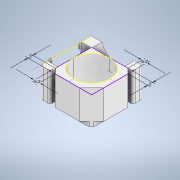
# Autodesk Inventor part: xy-mount-bottom-copy
Saved by Autodesk Inventor 2020 (Build 240168000, 168)
## iProperties
Created: 2021-03-01
Part Number: xy-mount-bottom-copy
Material: ABS Plastic
Document SubType Name: Modeling
Designer: AOB
Mass: 2.83472 g
Surface Area: 25.5195 cm^2
Volume: 2.67426 cm^3
Density: 1.06 g/cm^3
Appearance: White
Author: AOB
Autodesk Inventor part; units mm, degrees
ref_plane "YZ Plane" through (0, 0, 0) normal (1, 0, 0) x (0, 1, 0)
ref_plane "XZ Plane" through (0, 0, 0) normal (0, 1, 0) x (-1, 0, 0)
ref_plane "XY Plane" through (0, 0, 0) normal (0, 0, 1) x (1, 0, 0)
sketch "Sketch1" plane through (0, 0, 0) normal (0, 0, 1) x (1, 0, 0)
  line L0 (0, 0) -> (21, 0)
  line L1 (21, 0) -> (21, -24)
  line L2 (21, -24) -> (0, -24)
  line L3 (0, -24) -> (0, 0)
  line L4 (4, 0) -> (4, -24)
  line L5 (0, -24) -> (21, 0) construction
  line L6 (0, 0) -> (10.5, -12) construction
  dimension "d0" = 4
  dimension "d2" = 17
  dimension "d61" = 24
  constraints: 14 end point, 2 midpoint, 2 parallel, 2 perpendicular, 2 point on line, 1 horizontal
  measures "d0" distance of L0.start L4.start
  measures "d2" distance of L0.end L4.start
  measures "d61" distance of L0.end L1.end
extrude "Extrusion1" add sketch "Sketch1" along normal blind 17 contours L0 L4 L2 L3
extrude "Extrusion2" add sketch "Sketch1" against normal blind 4
sketch "Sketch2" plane through (0, 0, 0) normal (0, 0, 1) x (1, 0, 0)
  point P0 (0, 0)
  point P1 (11.0344, -10.0001)
hole "Hole1" at (11.0344, -10.0001, 0) direction (0, 0, -1) diameter 14 end through all
sketch "Sketch3" plane through (4, -24, 17) normal (1, 0, 0) x (0, 0, -1)
  line L0 (11.8812, 10.4951) -> (9.8812, 10.4951)
  point P0 (17, 24)
  constraints: 2 coincident, 2 end point, 4 other
hole "Hole2" at (4, -13.5049, 7.1188) direction (-1, 0, 0) diameter 14 end through all
fillet "Fillet2" radius 1 4 edges at (4, -12, 17) (0, -12, 17) (21, -12, 0) (21, -12, -4)
fillet "Fillet3" radius 0.1 1 edges at (4, -12, 0)
sketch "Sketch5" plane through (0, 0, -4) normal (0, 1, 0) x (1, 0, 0)
  line L0 (4, -4.1188) -> (4, -18.1188) projected
  line L1 (20, -4) -> (4.1, -4) construction
  line L2 (11.5, -4) -> (11.5, -11.5) construction
  line L3 (11.5, -11.5) -> (4, -11.5) construction
  circle A0 centre (11.5, -11.5) radius 7.5
  line L4 (11.5, -11.5) -> (15.8301, -4) construction
  line L5 (19, -11.5) -> (19.6263, -11.5) construction
  line L6 (15.8301, -4) -> (11.5, -4)
  line L7 (11.5, -11.5) -> (7.1699, -4) construction
  line L8 (7.1699, -4) -> (5.0048, -7.75)
  line L9 (11.5, -11.5) -> (2.8397, -11.5) construction
  line L10 (2.8397, -11.5) -> (5.0048, -15.25)
  line L11 (11.5, -11.5) -> (7.1699, -19)
  line L12 (7.1699, -19) -> (11.5, -19)
  line L13 (11.5, -11.5) -> (15.8301, -19) construction
  line L14 (15.8301, -19) -> (17.9952, -15.25)
  line L15 (11.5, -11.5) -> (20.1603, -11.5) construction
  line L16 (20.1603, -11.5) -> (17.9952, -7.75)
  line L17 (20.1603, -11.5) -> (17.9952, -15.25)
  line L18 (15.8301, -4) -> (17.9952, -7.75)
  line L19 (11.5, -4) -> (7.1699, -4)
  line L20 (2.8397, -11.5) -> (5.0048, -7.75)
  line L21 (7.1699, -19) -> (5.0048, -15.25)
  line L22 (15.8301, -19) -> (11.5, -19)
  point P0 (0, -4)
  point P1 (4, -4)
  point P2 (21, -4)
  dimension "d26" = 7.5
  dimension "d27" = 7.5
  dimension "d28" = 60
  dimension "d31" = 360
  constraints: 42 end point, 3 point on line, 3 tangent, 2 perpendicular, 2 point on circle, 1 centre point, 1 coincident, 1 horizontal, 1 parallel, 1 vertical, 31 other
  measures "d26" distance of L2.start L2.end
  measures "d27" distance of L2.end L3.end
  measures "d28" angle of L5 L4
ref_plane "Work Plane1" through (0, -12, -4) normal (0, 1, 0) x (1, 0, 0)
sketch "Sketch6" plane through (0, -12, -4) normal (0, 1, 0) x (1, 0, 0)
  circle A0 centre (11.5, -11.5) radius 7.5 projected
  line L0 (11.5, -19) -> (11.5, -21) construction
  line L1 (19, -11.5) -> (21, -11.5) construction
  line L2 (0, -20) -> (0, 0) projected
  line L3 (0, -25) -> (0, 0) construction
  line L4 (19, -4) -> (4, -4)
  line L5 (4, -4) -> (4, -19)
  line L6 (4, -4.1) -> (4, -20) projected
  line L7 (21, -21) -> (6, -21)
  line L8 (21, -6) -> (21, -21)
  arc A1 (4.1, -4) -> (4, -4.1) centre (4.1, -4.1) ccw projected
  line L9 (21, -6) -> (19, -4)
  line L10 (4, -19) -> (6, -21)
  point P0 (0, -4)
  point P1 (4, -11.5)
  point P2 (4, -11.5)
  point P3 (21, -4)
  point P4 (4, -21)
  point P5 (11.5, -4)
  dimension "d86" = 2
  dimension "d87" = 2
  dimension "d88" = 2
  dimension "d89" = 2
  constraints: 18 end point, 6 point on line, 2 horizontal, 2 point on circle, 1 perpendicular, 1 vertical
  measures "d86" distance of L8.start point (21, -4)
  measures "d87" distance of L4.start point (21, -4)
  measures "d88" distance of L5.end point (4, -21)
  measures "d89" distance of L7.end point (4, -21)
extrude "Extrusion3" add sketch "Sketch6" along normal mid plane 24
sketch "Sketch7" plane through (0, 0, -4) normal (0, 1, 0) x (1, 0, 0)
  circle A0 centre (11.5, -11.5) radius 7.5
  line L0 (4, -4) -> (19, -4)
  line L1 (19, -4) -> (19, -19)
  line L2 (19, -19) -> (4, -19)
  line L3 (4, -19) -> (4, -4)
  circle A1 centre (11.5, -11.5) radius 4.5
  point P0 (4, -11.5)
  point P1 (11.5, -4)
  dimension "d82" = 9
  constraints: 8 end point, 2 centre point, 2 parallel, 1 coincident, 1 horizontal, 1 perpendicular
  measures "d82" diameter of A1
extrude "Extrusion4" add sketch "Sketch7" along normal blind 2 contours A0 | L1 L2 A0 | A0 L0 L1 | L2 L3 A0
mirror "Mirror1" about plane through (0, -12, -4) normal (0, 1, 0) of "Extrusion4"
sketch "Sketch8" plane through (0, -24, -4) normal (-1, 0, 0) x (0, 0, 1)
  line L0 (18.0753, 23) -> (18.0753, -1)
  line L1 (16.4506, 11) -> (16.4506, 10)
  line L2 (16.4506, 10) -> (18.0753, 10)
  line L3 (18.0753, 10) -> (18.0753, 11)
  line L4 (18.0753, 11) -> (18.0753, 12)
  line L5 (16.4506, 12) -> (16.4506, 11)
  line L6 (16.4506, 12) -> (18.0753, 12)
  line L7 (3.1188, 11.5233) -> (3.1188, 9.5233)
  line L8 (3.1188, 9.5233) -> (4.7688, 9.5233)
  line L9 (4.7688, 9.5233) -> (4.7688, 11.5233)
  line L10 (4.7688, 11.5233) -> (3.1188, 11.5233)
  circle A0 centre (11.1188, 10.4951) radius 7 projected
  line L11 (20, 24) -> (20, 0) projected
  line L12 (18.1006, 11) -> (17.4506, 11) construction
  point P0 (4, 24)
  dimension "d44" = 0.65
  dimension "d45" = 1
  dimension "d65" = 0.65
  constraints: 24 end point, 4 perpendicular, 2 parallel, 1 horizontal, 1 midpoint, 1 point on line, 1 vertical, 2 other
  measures "d65" distance of L12.start L12.end
extrude "Extrusion5" add sketch "Sketch8" along normal blind 0.5 contours L0 L2 L1 L5 L6 A0 | A0 L6 L0 | A0 L10 L9 L8 | L8 L7 L10 A0
fillet "Fillet5" radius 2 2 edges at (-0.5, -13.4767, -0.8812) (-0.5, -13, 14.0753)
sketch "Sketch9" plane through (0, 0, -4) normal (0, 0, -1) x (-1, 0, 0)
  circle A0 centre (-11.0344, -10.0001) radius 7 projected
  line L0 (-4.0344, -10.0001) -> (-4.0344, -11.0001)
  line L1 (-4.0344, -11.0001) -> (-3.0344, -11.0001)
  line L2 (-3.0344, -9.0001) -> (-4.6844, -9.0001)
  line L3 (-4.6844, -9.0001) -> (-4.6844, -11.0001)
  line L4 (-4.0344, -11.0001) -> (-4.6844, -11.0001)
  line L5 (-3.0344, -11.0001) -> (-3.0344, -9.0001)
  line L6 (-17.9794, -10.8755) -> (-19.0344, -10.8755)
  line L7 (-19.0344, -22.2481) -> (-19.0344, 1.7519)
  line L8 (-19.0344, -8.8755) -> (-17.3974, -8.8755)
  line L9 (-17.3974, -8.8755) -> (-17.3974, -10.8755)
  line L10 (-17.3974, -10.8755) -> (-17.9794, -10.8755)
  line L11 (-19.0344, -10.8755) -> (-19.0344, -8.8755)
  point P0 (0, 0)
  dimension "d50" = 1
  dimension "d51" = 0.65
  dimension "d54" = 2
  dimension "d55" = 1
  dimension "d57" = 0.582
  dimension "d58" = 1.055
  constraints: 24 end point, 4 perpendicular, 4 point on line, 3 horizontal, 2 point on circle, 2 vertical, 1 tangent
  measures "d50" distance of L0.end L1.end
  measures "d51" distance of L0.end L3.end
  measures "d54" distance of L2.end L3.end
  measures "d55" distance of L0.start L0.end
  measures "d57" distance of L9.end L6.start
  measures "d58" distance of L6.start L6.end
chamfer "Chamfer2" distance 5 angle 45 1 edges at (21, -12, 17)
extrude "Extrusion6" add sketch "Sketch9" along normal blind 0.5 contours A0 L4 L3 L2 | L0 L4 A0 | A0 L2 L5 L1 L0 | L8 L9 L10 A0 | A0 L6 L7 L8
fillet "Fillet6" radius 2 2 edges at (19.0344, -9.8755, -4.5) (3.0344, -10.0001, -4.5)
split "Split1" plane through (0, -12, -4) removes the side toward (0, 1, 0)
hole "Hole5" at (11.5, -12, 7.5) direction (0, -1, 0) diameter 15 depth 12
body "Solid1"
